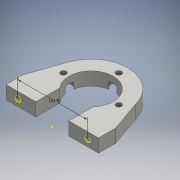
# Autodesk Inventor part: ROTATION2
Saved by Autodesk Inventor 2016 (Build 200138000, 138)
## iProperties
Created: 2017-07-15
Part Number: ROTATION2
Material: Generic
Document SubType Name: Modeling
Designer: ALIREZA
Density: 1 g/cm^3
Appearance: Default
Author: ALIREZA
Autodesk Inventor part; units mm, degrees
ref_plane "YZ Plane" through (0, 0, 0) normal (1, 0, 0) x (0, 1, 0)
ref_plane "XZ Plane" through (0, 0, 0) normal (0, 1, 0) x (-1, 0, 0)
ref_plane "XY Plane" through (0, 0, 0) normal (0, 0, 1) x (1, 0, 0)
sketch "Sketch1" plane through (0, 0, 0) normal (0, 0, 1) x (1, 0, 0)
  circle A0 centre (0, 0) radius 10
  arc A1 (13.1244, -10) -> (-13.1244, -10) centre (0, 0) ccw
  line L0 (13.1244, -10) -> (25, -10)
  line L1 (25, -10) -> (0, -10)
  line L2 (-13.1244, -10) -> (-25, -10)
  line L3 (0, 0) -> (0, -17.5)
  line L4 (0, -17.5) -> (-25, -17.5)
  line L5 (-25, -17.5) -> (-25, -10)
  line L6 (25, -10) -> (25, -17.5)
  line L7 (25, -17.5) -> (0, -17.5)
  line L8 (0, 0) -> (-12.5, 0)
  circle A2 centre (-12.5, 0) radius 1.25
  line L9 (0, 0) -> (0, 12.5)
  circle A3 centre (0, 12.5) radius 1.25
  circle A4 centre (12.5, 0) radius 1.25
  circle A5 centre (0, -12.5) radius 1.25
  circle A6 centre (12.5, 0) radius 3.25
  circle A7 centre (-12.5, 0) radius 3.25
  line L10 (0, 0) -> (2.11, 2.11)
  line L11 (0, 0) -> (2.984, 0) construction
  circle A8 centre (0, 12.5) radius 3.25
  circle A9 centre (0, -12.5) radius 3.25
  dimension "d0" = 20
  dimension "d1" = 33
  dimension "d2" = 25
  dimension "d3" = 25
  dimension "d4" = 17.5
  dimension "d5" = 25
  dimension "d6" = 12.5
  dimension "d7" = 2.5
  dimension "d8" = 12.5
  dimension "d9" = 2.5
  dimension "d15" = 6.5
  dimension "d16" = 45
  dimension "d17" = 6.5
  dimension "d18" = 6.5
  constraints: 24 end point, 9 centre point, 7 coincident, 6 horizontal, 3 perpendicular, 2 point on circle, 2 point on line, 2 symmetric about line, 2 vertical, 1 collinear, 1 equal length, 1 parallel, 1 vertical alignment, 5 other
  measures "d1" diameter of A1
  measures "d2" distance of L1.end L0.end
  measures "d3" distance of L1.end L2.end
  measures "d4" distance of L3.start L3.end
  measures "d5" distance between parallel lines of L3 L5
  measures "d6" distance of L3.start L8.end
  measures "d7" diameter of A2
  measures "d8" distance of L3.start L9.end
  measures "d9" diameter of A3
  measures "d15" diameter of A6
  measures "d16" angle of L11 L10
  measures "d17" diameter of A8
  measures "d18" diameter of A9
extrude "Extrusion1" add sketch "Sketch1" along normal blind 6 contours A0 A6 | A0 A8 A7 A9 L3 L4 L5 L2 A1 L1 A6 | A0 A8 | A9 L1 A0 | L3 A5 A9 A0 | L1 A9 L3 A5 | L1 L0 L6 L7 L3 A9 | A5 L3 | L3 A5 | A0 A7 picked at (10.6028, 1.4923)
fillet "Fillet1" radius 5 2 edges at (13.1244, -10, 3) (-13.1244, -10, 3)
sketch "Sketch2" plane through (0, 0, 0) normal (0, 0, -1) x (-1, 0, 0)
  circle A0 centre (0, 12.5) radius 1.25 projected
  line L0 (0, 0) -> (-3.0567, 0)
  circle A1 centre (0, -12.5) radius 1.25
  constraints: 2 end point, 1 centre point, 1 horizontal, 1 symmetric about line, 1 other
extrude "Extrusion2" cut sketch "Sketch2" against normal blind 10 contours A1
sketch "Sketch3" plane through (0, 0, 0) normal (0, 0, -1) x (-1, 0, 0)
  circle A0 centre (-12.5, 0) radius 1.25 projected
  circle A1 centre (0, -12.5) radius 1.25 projected
  circle A2 centre (0, 0) radius 10 projected
  circle A3 centre (-12.5, 0) radius 1.25 projected
  circle A4 centre (0, 12.5) radius 1.25 projected
  circle A5 centre (12.5, 0) radius 1.25 projected
  line L0 (25, -17.5) -> (-25, -17.5) projected
  line L1 (25, -10) -> (25, -17.5) projected
  line L2 (20.9105, -10) -> (25, -10) projected
  arc A6 (16.0476, -3.8372) -> (20.9105, -10) centre (20.9105, -5) ccw projected
  arc A7 (16.0476, -3.8372) -> (-16.0476, -3.8372) centre (0, 0) ccw projected
  arc A8 (-20.9105, -10) -> (-16.0476, -3.8372) centre (-20.9105, -5) ccw projected
  line L3 (-25, -10) -> (-20.9105, -10) projected
  line L4 (-25, -17.5) -> (-25, -10) projected
  circle A9 centre (-12.5, 0) radius 3.25
  circle A10 centre (0, 12.5) radius 3.25
  circle A11 centre (12.5, 0) radius 1.25 projected
  circle A12 centre (12.5, 0) radius 3.25
  circle A13 centre (0, -12.5) radius 3.25
  dimension "d19" = 6.5
  dimension "d20" = 6.5
  dimension "d21" = 6.5
  dimension "d22" = 6.5
  constraints: 4 centre point, 4 coincident
  measures "d19" diameter of A9
  measures "d20" diameter of A10
  measures "d21" diameter of A12
  measures "d22" diameter of A13
extrude "Extrusion3" cut sketch "Sketch3" against normal blind 3 contours A2 A12 | A2 A12 | A10 A2 | A2 A10 | A13 A2 | A2 A13 | A9 A2 | A2 A9
sketch "Sketch4" plane through (0, 0, 0) normal (0, 0, -1) x (-1, 0, 0)
  arc A0 (16.0476, -3.8372) -> (-16.0476, -3.8372) centre (0, 0) ccw projected
  line L0 (-25, -10) -> (-20.9105, -10) projected
  line L1 (-16.0476, 3.8372) -> (-20.9105, -10)
  line L2 (15.5959, 5.3868) -> (20.9105, -10)
  arc A1 (16.0476, -3.8372) -> (20.9105, -10) centre (20.9105, -5) ccw projected
  arc A2 (-20.9105, -10) -> (-16.0476, -3.8372) centre (-20.9105, -5) ccw projected
  constraints: 4 end point, 3 point on circle, 1 tangent
extrude "Extrusion4" add sketch "Sketch4" against normal up to surface (6 mm away)
sketch "Sketch5" plane through (-25, -17.5, 0) normal (0, -1, 0) x (1, 0, 0)
  line L0 (0, 6) -> (50, 6) projected
  line L1 (0, 0) -> (50, 0) projected
  circle A0 centre (40.75, 3) radius 1.25
  circle A1 centre (9.25, 3) radius 1.25
  point P0 (25, 0)
  dimension "d27" = 2.5
  constraints: 2 centre point
  measures "d27" diameter of A0
extrude "Extrusion5" cut sketch "Sketch5" against normal blind 14
sketch "Sketch6" plane through (-25, -17.5, 0) normal (0, -1, 0) x (1, 0, 0)
  circle A0 centre (9.25, 3) radius 1.25 projected
  circle A1 centre (40.75, 3) radius 1.25 projected
  point P0 (25, 0)
  dimension "d30" = 31.5
  measures "d30" distance of A0.centre A1.centre
sketch "Sketch7" plane through (-25, -17.5, 0) normal (0, -1, 0) x (1, 0, 0)
  line L0 (32.5, -8.9217) -> (17.5, -8.9217)
  line L1 (17.5, -8.9217) -> (17.5, 8.9217)
  line L2 (17.5, 8.9217) -> (32.5, 8.9217)
  line L3 (32.5, 8.9217) -> (32.5, -8.9217)
  line L4 (32.5, -8.9217) -> (17.5, 8.9217) construction
  line L5 (17.5, -8.9217) -> (32.5, 8.9217) construction
  point P0 (25, 0)
  dimension "d31" = 15
  constraints: 12 end point, 2 midpoint, 2 parallel, 1 horizontal, 1 perpendicular
  measures "d31" distance of L1.end L2.end
extrude "Extrusion6" cut sketch "Sketch7" against normal blind 14
sketch "Sketch8" plane through (-25, -10, 6) normal (0, 1, 0) x (1, 0, 0)
  line L0 (9.4041, 6) -> (41.0476, 6) projected
  line L1 (4.0895, 6) -> (4.0895, 0) projected
  line L2 (9.4041, 6) -> (4.0895, 6)
  line L3 (4.0895, 6) -> (4.0895, 0)
  line L4 (4.0895, 0) -> (9.4041, 0)
  line L5 (9.4041, 0) -> (9.4041, 6)
  line L6 (45.8371, 0) -> (50, 0)
  line L7 (50, 0) -> (50, 6)
  line L8 (50, 6) -> (45.8371, 6)
  line L9 (45.8371, 6) -> (45.8371, 0)
  line L10 (0, 0) -> (4.0895, 0)
  line L11 (4.0895, 0) -> (4.0895, 6)
  line L12 (4.0895, 6) -> (0, 6)
  line L13 (0, 6) -> (0, 0)
  point P0 (25, 6)
  constraints: 24 end point, 6 parallel, 3 horizontal, 3 perpendicular, 1 point on line
extrude "Extrusion7" cut sketch "Sketch8" against normal blind 14 contours L1 L10 L13 L12 | L9 L8 L7 L6
body "Solid1"
